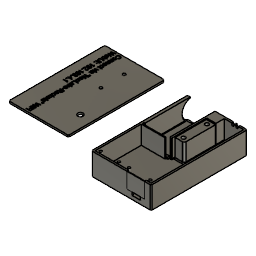
NeoLabs-Rocket-LaunchSystem (Autodesk Fusion 360 design; units mm, degrees)
part number: 2026-06-22-15-23-40-564
Autodesk Fusion 360 part; units mm, degrees
sketch "Sketch1" plane through (0, 0, 0) normal (0, 0, 1) x (1, 0, 0)
  line L0 (-60, -35) -> (5, -35)
  line L1 (5, -35) -> (5, 69.6198)
  line L2 (5, 69.6198) -> (-60, 69.6198)
  line L3 (-60, 69.6198) -> (-60, -35)
  circle A0 centre (-54.5, -30.5) radius 1.35
  circle A1 centre (-34.5, -30.5) radius 1.35
  circle A2 centre (-23.5, -30.5) radius 1.35
  circle A3 centre (-0.5, -30.5) radius 1.35
  dimension "d1" = 65
  dimension "d9" = 2.7
  dimension "d10" = 2.7
  dimension "d11" = 2.7
  dimension "d12" = 2.7
  constraint horizontal L0
  constraint vertical L1
  constraint horizontal L2
  constraint vertical L3
  measures "d1" distance of L0.start L0.end
  measures "d9" diameter of A0
  measures "d10" diameter of A1
  measures "d11" diameter of A2
  measures "d12" diameter of A3
extrude "Extrude1" add sketch "Sketch1" against normal blind 4 makes body 1
extrude "Extrude2" add sketch "Sketch1" along normal blind 6 and the other way blind 4 contours A0 | A1 | A2 | A3 bodies 1
sketch "Sketch2" plane through (0, 0, 0) normal (0, 0, 1) x (-1, 0, 0)
  line L0 (60, -69.6198) -> (60, 35)
  line L1 (60, 35) -> (-5, 35)
  line L2 (-5, 35) -> (-5, -69.6198)
  line L3 (-5, -69.6198) -> (60, -69.6198)
  circle A0 centre (0.5, 30.5) radius 1.35
  circle A1 centre (34.5, 30.5) radius 1.35
  circle A2 centre (54.5, 30.5) radius 1.35
  circle A3 centre (23.5, 30.5) radius 1.35
  line L4 (30.3925, -68.4602) -> (56.3925, -68.4602)
  line L5 (56.3925, -68.4602) -> (56.3925, -20.4602)
  line L6 (56.3925, -20.4602) -> (30.3925, -20.4602)
  line L7 (30.3925, -20.4602) -> (30.3925, -68.4602)
  line L8 (31.8289, -17.2317) -> (57.8727, -17.2317)
  line L9 (57.8727, -17.2317) -> (57.8727, -18.2915)
  line L10 (57.8727, -18.2915) -> (31.8289, -18.2915)
  line L11 (31.8289, -18.2915) -> (31.8289, -17.2317)
  line L12 (57.8615, -18.2915) -> (57.8615, -20.4602)
  line L13 (31.8289, -20.7915) -> (31.8289, -21.7915)
  line L14 (59.9993, -21.7915) -> (59.9993, -16.2915)
  line L15 (57.8615, -17.2317) -> (57.8615, -20.4602)
  line L16 (60, -69.6198) -> (58, -69.6198)
  line L17 (60, -21.7915) -> (60, -69.6198)
  line L18 (60, -21.7915) -> (59.9993, -21.7915)
  line L19 (57.9993, -16.2915) -> (57.9993, 33)
  line L20 (57.9993, 35) -> (59.9993, 35)
  line L21 (59.9993, 35) -> (59.9993, -16.2915)
  line L22 (-5, 35) -> (-3, 35)
  line L23 (-3, 33) -> (-3, -67.6198)
  line L24 (-3, -69.6198) -> (-5, -69.6198)
  line L25 (-5, -69.6198) -> (-5, 35)
  line L26 (-3, -69.6198) -> (30.1003, -69.6198)
  line L27 (30.1003, -69.6198) -> (30.1003, -67.6198)
  line L28 (17.9963, -67.6198) -> (-3, -67.6198)
  line L29 (58, -69.6198) -> (56.8045, -69.6198)
  line L30 (56.8045, -69.6198) -> (56.8045, -67.6198)
  line L31 (30.3925, -20.4602) -> (57.8727, -20.4602)
  line L32 (57.8727, -20.4602) -> (57.8727, -18.2915)
  line L33 (57.8727, -18.2915) -> (30.3925, -18.2915)
  line L34 (30.3925, -18.2915) -> (30.3925, -20.4602)
  line L35 (-5, 35) -> (60, 35)
  line L36 (60, 35) -> (60, 33)
  line L37 (-5, 33) -> (-5, 35)
  line L38 (60, 33) -> (59.9993, 33)
  line L39 (57.9993, 33) -> (-3, 33)
  line L40 (28.1003, -58.5213) -> (28.1003, -20.4602)
  line L41 (28.1003, -20.4602) -> (30.1003, -20.4602)
  line L42 (30.1003, -20.4602) -> (30.1003, -67.6198)
  line L43 (57.8727, -20.4602) -> (56.8045, -20.4602)
  line L44 (56.8045, -20.4602) -> (56.8045, -67.6198)
  line L45 (28.1003, -58.5213) -> (17.9963, -58.5213)
  line L46 (17.9963, -58.5213) -> (17.9963, -67.6198)
  line L47 (57.9993, -16.2915) -> (57.9993, -17.2317)
  line L48 (57.9993, -17.2317) -> (57.8727, -17.2317)
  dimension "d27" = 26
  dimension "d28" = 48
  dimension "d34" = 2
  dimension "d35" = 2
  dimension "d36" = 2
  dimension "d37" = 2
  constraint horizontal L4
  constraint vertical L5
  constraint horizontal L6
  constraint vertical L7
  constraint horizontal L8
  constraint vertical L9
  constraint horizontal L10
  constraint vertical L11
  constraint coincident L10 L12.start
  constraint perpendicular L10 L12
  constraint vertical L13
  constraint vertical L14
  constraint vertical L15
  constraint horizontal L16
  constraint vertical L17
  constraint coincident L0.start L3.end
  constraint vertical L19
  constraint horizontal L20
  constraint vertical L21
  constraint horizontal L22
  constraint vertical L23
  constraint horizontal L24
  constraint vertical L25
  constraint coincident L1.end L2.start
  constraint horizontal L26
  constraint vertical L27
  constraint horizontal L28
  constraint horizontal L29
  constraint vertical L30
  constraint horizontal L31
  constraint vertical L32
  constraint horizontal L33
  constraint vertical L34
  constraint horizontal L35
  constraint vertical L36
  constraint horizontal L38
  constraint vertical L37
  constraint coincident L0 L36.end
  constraint coincident L21 L38.end
  constraint collinear L38 L39
  constraint vertical L40
  constraint horizontal L41
  constraint vertical L42
  constraint horizontal L43
  constraint vertical L44
  constraint coincident L31 L12.end
  constraint horizontal L45
  constraint vertical L46
  constraint perpendicular L8 L47
  constraint perpendicular L15 L48
  constraint coincident L8 L15.start
  measures "d27" distance of L4.start L4.end
  measures "d28" distance of L4.start L6.end
  measures "d34" distance of L0.start L16.end
  measures "d35" distance of L14.end L19.start
  measures "d36" distance of L1.end L22.end
  measures "d37" distance of L24.start L23.end
extrude "Extrude3" add sketch "Sketch2" along normal blind 10 contours L8 L10 L11 L15 L33 bodies 1
extrude "Extrude5" add sketch "Sketch2" along normal blind 2 contours L6 L10 L12 L15 L31 L33 L34 L43 bodies 1
extrude "Extrude6" add sketch "Sketch2" along normal blind 20 contours L0 L1 L2 L3 L9 L14 L16 L17 L19 L20 L21 L22 L23 L24 L25 L26 L27 L28 L29 L30 L31 L32 L35 L36 L37 L39 L40 L41 L42 L43 L44 L45 L46 L47 L48 | L10 L12 L15 L31 L32 L33 L43 | L8 L9 L10 L15 L33 | L8 L10 L11 L15 L33 | A0 | A1 | A2 | A3 bodies 1
sketch "Sketch3" plane through (0, 0, 20) normal (0, 0, 1) x (-1, 0, 0)
  line L0 (56.8045, -69.6198) -> (60, -69.6198)
  line L1 (60, -69.6198) -> (60, -21.7915)
  line L2 (60, -21.7915) -> (59.9993, -21.7915)
  line L3 (59.9993, -21.7915) -> (59.9993, 35)
  line L4 (59.9993, 35) -> (-5, 35)
  line L5 (-5, 35) -> (-5, -69.6198)
  line L6 (9.8858, -69.6198) -> (7.3858, -69.6198)
  line L7 (7.3858, -69.6198) -> (7.3858, -67.6198)
  line L8 (7.3858, -67.6198) -> (9.8858, -67.6198)
  line L9 (9.8858, -67.6198) -> (9.8858, -69.6198)
  line L10 (5.5599, -69.6198) -> (3.0599, -69.6198)
  line L11 (3.0599, -69.6198) -> (3.0599, -67.6198)
  line L12 (3.0599, -67.6198) -> (5.5599, -67.6198)
  line L13 (5.5599, -67.6198) -> (5.5599, -69.6198)
  line L14 (57.8615, -18.2915) -> (31.8289, -18.2915)
  line L15 (31.8289, -18.2915) -> (31.8289, -17.2915)
  line L16 (31.8289, -17.2915) -> (57.8615, -17.2915)
  line L17 (57.8615, -17.2915) -> (57.8615, -18.2915)
  line L18 (57.9993, -16.2915) -> (57.9993, -17.2915)
  line L19 (57.8615, -17.2915) -> (57.9993, -17.2915)
  line L20 (57.9993, 33) -> (57.9993, -17.2317)
  line L21 (31.8289, -17.2317) -> (31.8289, -18.2915)
  line L22 (31.8289, -18.2915) -> (57.8615, -18.2915)
  line L23 (57.8615, -18.2915) -> (57.8615, -20.4602)
  line L24 (57.8615, -20.4602) -> (56.8045, -20.4602)
  line L25 (56.8045, -20.4602) -> (56.8045, -69.6198)
  line L26 (-5, -69.6198) -> (30.1003, -69.6198)
  line L27 (30.1003, -69.6198) -> (30.1003, -20.4602)
  line L28 (30.1003, -20.4602) -> (28.1003, -20.4602)
  line L29 (28.1003, -20.4602) -> (28.1003, -58.5213)
  line L30 (28.1003, -58.5213) -> (17.9963, -58.5213)
  line L31 (17.9963, -58.5213) -> (17.9963, -67.6198)
  line L32 (17.9963, -67.6198) -> (-3, -67.6198)
  line L33 (-3, -67.6198) -> (-3, 33)
  line L34 (-3, 33) -> (57.9993, 33)
  dimension "d48" = 2.5
  dimension "d49" = 2.5
  constraint horizontal L6
  constraint vertical L7
  constraint horizontal L8
  constraint vertical L9
  constraint horizontal L10
  constraint vertical L11
  constraint horizontal L12
  constraint vertical L13
  constraint horizontal L14
  constraint vertical L15
  constraint horizontal L16
  constraint vertical L17
  constraint perpendicular L18 L19
  measures "d48" distance of L6.start L6.end
  measures "d49" distance of L10.start L10.end
extrude "Extrude7" cut sketch "Sketch3" against normal blind 2.5 contours L10 L11 L12 L13 L26 L32 | L6 L7 L8 L9 L26 L32 bodies 1
fillet "Fillet1" radius 1 4 edges at (-3.0599, 68.6198, 17.5) (-5.5599, 68.6198, 17.5) (-9.8858, 68.6198, 17.5) (-7.3858, 68.6198, 17.5) on bodies 1
sketch "Sketch4" plane through (-60, 0, 0) normal (-1, 0, 0) x (0, -1, 0)
  line L0 (-69.6198, 20) -> (-69.6198, -4)
  line L1 (-69.6198, -4) -> (35, -4)
  line L2 (35, -4) -> (35, 0)
  line L3 (35, 0) -> (-21.7915, 0)
  line L4 (-21.7915, 0) -> (-21.7915, 20)
  line L5 (-21.7915, 20) -> (-69.6198, 20)
  circle A0 centre (-72, 8) radius 10.4908
extrude "Extrude8" cut sketch "Sketch4" against normal blind 38 contours L0 A0 | L0 A0 bodies 1
fillet "Fillet2" radius 1 6 edges at (-22, 69.6198, 8) (-26.0501, 69.6198, 18.2172) (-41, 69.6198, -2.2172) (-58.4022, 69.6198, 18.2172) (-30.1003, 61.8033, 10.4663) (-56.8045, 61.8033, 10.4663) on bodies 1
sketch "Sketch5" plane through (0, 0, 0) normal (0, 0, 1) x (-1, 0, 0)
  line L0 (6.8, 32.85) -> (15.8, 32.85)
  line L1 (15.8, 32.85) -> (6.8, 32.85)
  line L2 (6.8, 32.85) -> (6.8, 37.441)
  line L3 (6.8, 37.441) -> (15.8, 37.441)
  line L4 (15.8, 37.441) -> (15.8, 32.85)
  circle A0 centre (54.5, 30.5) radius 1.35
  circle A1 centre (34.5, 30.5) radius 1.35
  circle A2 centre (0.5, 30.5) radius 1.35
  circle A3 centre (23.5, 30.5) radius 1.35
  line L5 (29.1003, -65.2135) -> (57.8045, -65.2135)
  spline S0 degree 3 poles (57.8045, -65.2135) (57.6964, -65.2135) (57.5714, -65.179) (57.3554, -65.0637) (57.235, -64.9522) (57.0463, -64.708) (56.9546, -64.5234) (56.8406, -64.1757) (56.8045, -63.9456) (56.8045, -63.7515) knots 0.358129 0.358129 0.358129 0.358129 0.39055 0.39055 0.431579 0.431579 0.483124 0.483124 0.541351 0.541351 0.541351 0.541351
  line L6 (56.8045, -63.7515) -> (56.8045, -20.4602)
  line L7 (56.8045, -20.4602) -> (30.3925, -20.4602)
  line L8 (30.3925, -20.4602) -> (30.3925, -18.2915)
  line L9 (30.3925, -18.2915) -> (31.8289, -18.2915)
  line L10 (31.8289, -18.2915) -> (31.8289, -17.2317)
  line L11 (31.8289, -17.2317) -> (57.9993, -17.2317)
  line L12 (57.9993, -17.2317) -> (57.9993, 33)
  line L13 (57.9993, 33) -> (-3, 33)
  line L14 (-3, 33) -> (-3, -67.6198)
  line L15 (-3, -67.6198) -> (17.9963, -67.6198)
  line L16 (17.9963, -67.6198) -> (17.9963, -58.5213)
  line L17 (17.9963, -58.5213) -> (28.1003, -58.5213)
  line L18 (28.1003, -58.5213) -> (28.1003, -20.4602)
  line L19 (28.1003, -20.4602) -> (30.1003, -20.4602)
  line L20 (30.1003, -20.4602) -> (30.1003, -63.7515)
  spline S1 degree 3 poles (30.1003, -63.7515) (30.1003, -63.9456) (30.0641, -64.1757) (29.9501, -64.5234) (29.8585, -64.708) (29.6697, -64.9522) (29.5493, -65.0637) (29.3333, -65.179) (29.2083, -65.2135) (29.1003, -65.2135) knots 0.174906 0.174906 0.174906 0.174906 0.233133 0.233133 0.284679 0.284679 0.325708 0.325708 0.358129 0.358129 0.358129 0.358129
  dimension "d60" = 9
  constraint horizontal L1
  constraint vertical L2
  constraint horizontal L3
  constraint vertical L4
  measures "d60" distance of L0.start L0.end
extrude "Extrude9" cut sketch "Sketch5" along normal blind 3.2 contours L2 L3 L4 L13 bodies 1
sketch "Sketch6" plane through (0, 0, 20) normal (0, 0, 1) x (-1, 0, 0)
  line L0 (3.0599, -69.6198) -> (3.0599, -67.6198)
  line L1 (56.8045, -69.6198) -> (60, -69.6198)
  line L2 (60, -69.6198) -> (60, -21.7915)
  line L3 (60, -21.7915) -> (59.9993, -21.7915)
  line L4 (59.9993, -21.7915) -> (59.9993, 35)
  line L5 (59.9993, 35) -> (-5, 35)
  line L6 (-5, 35) -> (-5, -69.6198)
  line L7 (21.6224, 33) -> (2.3035, 33)
  line L8 (2.3035, 33) -> (2.3035, 34.4706)
  line L9 (2.3035, 34.4706) -> (21.6224, 34.4706)
  line L10 (21.6224, 34.4706) -> (21.6224, 33)
  line L11 (3.0599, -67.6198) -> (-3, -67.6198)
  line L12 (-3, -67.6198) -> (-3, 33)
  line L13 (-3, 33) -> (57.9993, 33)
  line L14 (57.9993, 33) -> (57.9993, -17.2317)
  line L15 (57.9993, -17.2317) -> (31.8289, -17.2317)
  line L16 (31.8289, -17.2317) -> (31.8289, -18.2915)
  line L17 (31.8289, -18.2915) -> (57.8615, -18.2915)
  line L18 (57.8615, -18.2915) -> (57.8615, -20.4602)
  line L19 (57.8615, -20.4602) -> (56.8045, -20.4602)
  line L20 (56.8045, -20.4602) -> (56.8045, -69.6198)
  line L21 (-5, -69.6198) -> (3.0599, -69.6198)
  constraint horizontal L7
  constraint vertical L8
  constraint horizontal L9
  constraint vertical L10
extrude "Extrude10" cut sketch "Sketch6" against normal blind 17 contours L7 L8 L9 L10 L13 bodies 1
fillet "Fillet3" radius 0.5 4 edges at (-1.7586, -30.0118, 0) (-24.7586, -30.0118, 0) (-35.7586, -30.0118, 0) (-55.7586, -30.0118, 0) on bodies 1
sketch "Sketch7" plane through (0, 0, 0) normal (0, 0, 1) x (-1, 0, 0)
  circle A0 centre (34.5, 30.5) radius 1.85
  circle A1 centre (0.5, 30.5) radius 1.85
  line L0 (29.1003, -65.2135) -> (57.8045, -65.2135)
  spline S0 degree 3 poles (57.8045, -65.2135) (57.6964, -65.2135) (57.5714, -65.179) (57.3554, -65.0637) (57.235, -64.9522) (57.0463, -64.708) (56.9546, -64.5234) (56.8406, -64.1757) (56.8045, -63.9456) (56.8045, -63.7515) knots 0.358129 0.358129 0.358129 0.358129 0.39055 0.39055 0.431579 0.431579 0.483124 0.483124 0.541351 0.541351 0.541351 0.541351
  line L1 (56.8045, -63.7515) -> (56.8045, -20.4602)
  line L2 (56.8045, -20.4602) -> (30.3925, -20.4602)
  line L3 (30.3925, -20.4602) -> (30.3925, -18.2915)
  line L4 (30.3925, -18.2915) -> (31.8289, -18.2915)
  line L5 (31.8289, -18.2915) -> (31.8289, -17.2317)
  line L6 (31.8289, -17.2317) -> (57.9993, -17.2317)
  line L7 (57.9993, -17.2317) -> (57.9993, 33)
  line L8 (57.9993, 33) -> (15.8, 33)
  line L9 (15.8, 33) -> (15.8, 35)
  line L10 (15.8, 35) -> (6.8, 35)
  line L11 (6.8, 35) -> (6.8, 33)
  line L12 (6.8, 33) -> (-3, 33)
  line L13 (-3, 33) -> (-3, -67.6198)
  line L14 (-3, -67.6198) -> (17.9963, -67.6198)
  line L15 (17.9963, -67.6198) -> (17.9963, -58.5213)
  line L16 (17.9963, -58.5213) -> (28.1003, -58.5213)
  line L17 (28.1003, -58.5213) -> (28.1003, -20.4602)
  line L18 (28.1003, -20.4602) -> (30.1003, -20.4602)
  line L19 (30.1003, -20.4602) -> (30.1003, -63.7515)
  spline S1 degree 3 poles (30.1003, -63.7515) (30.1003, -63.9456) (30.0641, -64.1757) (29.9501, -64.5234) (29.8585, -64.708) (29.6697, -64.9522) (29.5493, -65.0637) (29.3333, -65.179) (29.2083, -65.2135) (29.1003, -65.2135) knots 0.174906 0.174906 0.174906 0.174906 0.233133 0.233133 0.284679 0.284679 0.325708 0.325708 0.358129 0.358129 0.358129 0.358129
  circle A2 centre (23.5, 30.5) radius 1.85
  circle A3 centre (54.5, 30.5) radius 1.85
  circle A4 centre (22.12, -52.8277) radius 2.05
  line L20 (27, -57) -> (17, -57)
  line L21 (17, -57) -> (17, -23)
  line L22 (17, -23) -> (27, -23)
  line L23 (27, -23) -> (27, -57)
  circle A5 centre (22.0931, -27.4434) radius 2.05
  dimension "d67" = 4.1
  dimension "d70" = 4.1
  constraint horizontal L20
  constraint vertical L21
  constraint horizontal L22
  constraint vertical L23
  measures "d67" diameter of A4
  measures "d70" diameter of A5
extrude "Extrude11" add sketch "Sketch7" along normal blind 20 contours L20 L21 L22 L23 bodies 1
extrude "Extrude12" add sketch "Sketch7" along normal blind 14 contours A4 | A5 bodies 1
fillet "Fillet4" radius 2 1 edges at (-17, 23, 10) on bodies 1
fillet "Fillet5" radius 0.5 4 edges at (-30.1003, 20.4602, 10) (-31.8289, 18.2915, 11) (-31.8289, 17.2317, 10) (-28.1003, 20.4602, 10) on bodies 1
fillet "Fillet6" radius 0.25 1 edges at (-30.3925, 18.2915, 1) on bodies 1
fillet "Fillet7" radius 1 3 edges at (-17, 41, 0) (-17.5858, 23.5858, 0) (-23, 23, 0) on bodies 1
fillet "Fillet8" radius 0.5 8 edges at (-57.0463, 64.6852, 0) (-56.8045, 42.1058, 0) (-28.1003, 39.7407, 0) (-28.2467, 20.6066, 0) (-29.1003, 20.4602, 0) (-29.9538, 20.6066, 0) (-30.1003, 42.3558, 0) (-29.8584, 64.6852, 0) on bodies 1
chamfer "Chamfer1" distance 1 angle 45 9 edges at (5, -35, 8) (5, 69.6198, 8) (-59.9993, -35, 10) (-60, -35, -2) (-60, 69.6198, 19.4912) (-60, 69.4242, 18.3883) (-60, 61.5092, 8) (-60, 69.4242, -2.3883) (-60, 69.6198, -3.4912) on bodies 1
sketch "Sketch8" plane through (0, 0, -4) normal (0, 0, -1) x (1, 0, 0)
  line L0 (-59, 35) -> (-60, 34)
  line L1 (-60, 34) -> (-60, -68.6198)
  line L2 (-60, -68.6198) -> (-59, -69.6198)
  line L3 (-59, -69.6198) -> (4, -69.6198)
  line L4 (4, -69.6198) -> (5, -68.6198)
  line L5 (5, -68.6198) -> (5, 34)
  line L6 (5, 34) -> (4, 35)
  line L7 (4, 35) -> (-59, 35)
  line L8 (-29.0162, -60) -> (-29.0162, 26.9173) construction
  line L9 (-29.0162, 26.9173) -> (-29.6831, 26.9173) construction
  line L10 (-29.6831, 26.9173) -> (-29.6831, -60) construction
  line L11 (-29.6831, -60) -> (-29.0162, -60) construction
  dimension "d84" = 10
  text T0 "NeoLabs\nLaunch-System" font "Arial" height 10 align centre middle in box 86.9173 x 0.6668 at (-29.0162, -60) x (0, 1) y (-1, 0) spacing 1 kerned
extrude "Extrude13" cut sketch "Sketch8" against normal blind 1 text T0 bodies 1
sketch "Sketch9" plane through (0, 0, 0) normal (0, 0, 1) x (-1, 0, 0)
  line L0 (27, -22) -> (27, -57)
  line L1 (27, -57) -> (16, -57)
  line L2 (16, -57) -> (16, -25)
  arc A0 (19, -22) -> (16, -25) centre (19, -25) ccw
  line L3 (19, -22) -> (27, -22)
  circle A1 centre (54.5, 30.5) radius 1.85
  circle A2 centre (23.5, 30.5) radius 1.85
  line L4 (27.6003, -58.5213) -> (27.6003, -20.9602)
  arc A3 (28.6003, -19.9602) -> (27.6003, -20.9602) centre (28.6003, -20.9602) ccw
  line L5 (28.6003, -19.9602) -> (29.6003, -19.9602)
  arc A4 (30.3925, -20.3499) -> (29.6003, -19.9602) centre (29.6003, -20.9602) ccw
  line L6 (30.3925, -20.3499) -> (30.3925, -18.5415)
  arc A5 (30.6425, -18.2915) -> (30.3925, -18.5415) centre (30.6425, -18.5415) ccw
  line L7 (30.6425, -18.2915) -> (31.8289, -18.2915)
  line L8 (31.8289, -18.2915) -> (31.8289, -17.7317)
  arc A6 (32.3289, -17.2317) -> (31.8289, -17.7317) centre (32.3289, -17.7317) ccw
  line L9 (32.3289, -17.2317) -> (57.9993, -17.2317)
  line L10 (57.9993, -17.2317) -> (57.9993, 33)
  line L11 (57.9993, 33) -> (15.8, 33)
  line L12 (15.8, 33) -> (15.8, 35)
  line L13 (15.8, 35) -> (6.8, 35)
  line L14 (6.8, 35) -> (6.8, 33)
  line L15 (6.8, 33) -> (-3, 33)
  line L16 (-3, 33) -> (-3, -67.6198)
  line L17 (-3, -67.6198) -> (17.9963, -67.6198)
  line L18 (17.9963, -67.6198) -> (17.9963, -58.5213)
  line L19 (17.9963, -58.5213) -> (27.6003, -58.5213)
  circle A7 centre (0.5, 30.5) radius 1.85
  circle A8 centre (34.5, 30.5) radius 1.85
  line L20 (10.6673, -61.4434) -> (10.6673, -26.1703) construction
  line L21 (10.6673, -26.1703) -> (0.8534, -26.1703) construction
  line L22 (0.8534, -26.1703) -> (0.8534, -61.4434) construction
  line L23 (0.8534, -61.4434) -> (10.6673, -61.4434) construction
  dimension "d88" = 5
  text T0 "Made by Neo" font "Arial" height 5 align centre middle in box 35.273 x 9.8139 at (10.6673, -61.4434) x (0, 1) y (-1, 0) spacing 1 kerned
extrude "Extrude14" cut sketch "Sketch9" against normal blind 1 text T0 bodies 1
sketch "Sketch10" plane through (0, 0, 20) normal (0, 0, 1) x (-1, 0, 0)
  line L0 (59, -69.6198) -> (60, -68.6198)
  line L1 (60, -68.6198) -> (60, -21.7915)
  line L2 (60, -21.7915) -> (59.9993, -21.7915)
  line L3 (59.9993, -21.7915) -> (59.9993, 34)
  line L4 (59.9993, 34) -> (58.9993, 35)
  line L5 (58.9993, 35) -> (-4, 35)
  line L6 (-4, 35) -> (-5, 34)
  line L7 (-5, 34) -> (-5, -68.6198)
  line L8 (-5, -68.6198) -> (-4, -69.6198)
  line L9 (-4, -69.6198) -> (3.0599, -69.6198)
  line L10 (3.0599, -69.6198) -> (3.0599, -67.6198)
  line L11 (3.0599, -67.6198) -> (-3, -67.6198)
  line L12 (-3, -67.6198) -> (-3, 33)
  line L13 (-3, 33) -> (2.3035, 33)
  line L14 (2.3035, 33) -> (2.3035, 34.4706)
  line L15 (2.3035, 34.4706) -> (21.6224, 34.4706)
  line L16 (21.6224, 34.4706) -> (21.6224, 33)
  line L17 (21.6224, 33) -> (57.9993, 33)
  line L18 (57.9993, 33) -> (57.9993, -17.2317)
  line L19 (57.9993, -17.2317) -> (32.3289, -17.2317)
  arc A0 (32.3289, -17.2317) -> (31.8289, -17.7317) centre (32.3289, -17.7317) ccw
  line L20 (31.8289, -17.7317) -> (31.8289, -17.7915)
  arc A1 (31.8289, -17.7915) -> (32.3289, -18.2915) centre (32.3289, -17.7915) ccw
  line L21 (32.3289, -18.2915) -> (57.8615, -18.2915)
  line L22 (57.8615, -18.2915) -> (57.8615, -20.4602)
  line L23 (57.8615, -20.4602) -> (56.8045, -20.4602)
  line L24 (56.8045, -20.4602) -> (56.8045, -69.6198)
  line L25 (56.8045, -69.6198) -> (59, -69.6198)
  line L26 (-4, 35) -> (58.9993, 35)
  line L27 (60, -21.7915) -> (60, -68.6198)
  line L28 (59, -69.6198) -> (-4, -69.6198)
  line L29 (59, -69.6198) -> (60, -68.6198)
  line L30 (-5, -68.6198) -> (-4, -69.6198)
  line L31 (-5, 34) -> (-4, 35)
  line L32 (58.9993, 35) -> (59.9993, 34)
  circle A2 centre (22.1319, -52.8525) radius 1.5
  circle A3 centre (22.1001, -27.462) radius 1.5
  circle A4 centre (8, 9) radius 2.8806
  dimension "d92" = 3
  dimension "d96" = 3
  constraint horizontal L26
  constraint vertical L27
  constraint horizontal L28
  constraint coincident L0.start L25.end
  constraint coincident L0.end L1.start
  constraint coincident L7.end L8.start
  constraint coincident L8.end L9.start
  constraint coincident L6.end L7.start
  constraint coincident L5.end L6.start
  constraint coincident L4.end L5.start
  constraint coincident L3.end L4.start
  measures "d92" diameter of A2
  measures "d96" diameter of A3
extrude "Extrude15" add sketch "Sketch10" along normal blind 2 separate body makes body 2
move_body "Move1" bodies 2 to x (1, 0, 0) y (0, 1, 0) z (0, 0, 1) at (-90, 0, 0)
sketch "Sketch11" plane through (0, 0, 22) normal (0, 0, 1) x (-1, 0, 0)
  circle A0 centre (112.1001, -27.462) radius 1.5
  circle A1 centre (112.1319, -52.8525) radius 1.5
  circle A2 centre (98, 9) radius 2.8806
  line L0 (85, 34) -> (85, -68.6198)
  line L1 (85, -68.6198) -> (86, -69.6198)
  line L2 (86, -69.6198) -> (149, -69.6198)
  line L3 (149, -69.6198) -> (150, -68.6198)
  line L4 (150, -68.6198) -> (150, -21.7915)
  line L5 (150, -21.7915) -> (149.9993, -21.7915)
  line L6 (149.9993, -21.7915) -> (149.9993, 34)
  line L7 (149.9993, 34) -> (148.9993, 35)
  line L8 (148.9993, 35) -> (86, 35)
  line L9 (86, 35) -> (85, 34)
  line L10 (149.4447, -67.9375) -> (148.9993, 35) construction
  line L11 (148.9993, 35) -> (120.1099, 34.875) construction
  line L12 (120.1099, 34.875) -> (120.5553, -68.0625) construction
  line L13 (120.5553, -68.0625) -> (149.4447, -67.9375) construction
  dimension "d97" = 4.4
  text T0 "Connect via \"NeoLabs-Rockets\" WiFi\nWebUI: 192.168.4.1" font "Arial" height 4.4 align left middle in box 102.9385 x 28.8896 at (149.4447, -67.9375) x (-0.004327, 0.999991) y (-0.999991, -0.004327) spacing 1 kerned
  constraint coincident L7.end
extrude "Extrude16" cut sketch "Sketch11" against normal blind 1 text T0 bodies 2
equation "d85 = 'NeoLabs Launch-System'"
equation "d89 = 'Made by Neo'"
equation "d98 = 'Connect via \"NeoLabs-Rockets\" WiFi WebUI: 192.168.4.1'"
